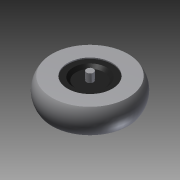
# Autodesk Inventor part: caster wheel
Saved by Autodesk Inventor 2012 (Build 160160000, 160)
## iProperties
Created: 2012-03-07
Part Number: caster wheel
Material: Default
Document SubType Name: Modeling
Designer: esv
Density: 1 g/cm^3
Author: esv
Autodesk Inventor part; units mm, degrees
ref_plane "YZ Plane" through (0, 0, 0) normal (1, 0, 0) x (0, 1, 0)
ref_plane "XZ Plane" through (0, 0, 0) normal (0, 1, 0) x (-1, 0, 0)
ref_plane "XY Plane" through (0, 0, 0) normal (0, 0, 1) x (1, 0, 0)
sketch "Sketch1" plane through (0, 0, 0) normal (0, 0, 1) x (1, 0, 0)
  line L0 (0, 0) -> (0, 0)
  line L1 (95.25, 0) -> (95.25, 7.7978)
  line L2 (86.36, -27.94) -> (50.8, -27.94)
  line L3 (50.8, -27.94) -> (50.8, 27.94)
  line L4 (50.8, 27.94) -> (86.36, 27.94)
  line L5 (86.36, 27.94) -> (86.36, -27.94)
  line L6 (50.8, 25.4) -> (38.1, 25.4)
  line L7 (38.1, 25.4) -> (38.1, -25.4)
  line L8 (38.1, -25.4) -> (50.8, -25.4)
  line L9 (50.8, -25.4) -> (50.8, 25.4)
  line L10 (0, 19.05) -> (31.75, 19.05)
  line L11 (31.75, 19.05) -> (31.75, -19.05)
  line L12 (31.75, -19.05) -> (0, -19.05)
  line L13 (0, -19.05) -> (0, 19.05)
  line L14 (31.75, 19.05) -> (38.1, 25.4)
  line L15 (38.1, -25.4) -> (31.75, -19.05)
  line L16 (0, 7.7978) -> (4.1037, 7.7978)
  line L17 (0, 38.1) -> (7.9375, 38.1)
  line L18 (7.9375, 38.1) -> (7.9375, -38.1)
  line L19 (7.9375, -38.1) -> (0, -38.1)
  line L20 (0, -38.1) -> (0, 38.1)
  arc A0 (86.36, -27.94) -> (86.36, 27.94) centre (46.8993, 0) ccw
  point P0 (50.8, 0)
  point P1 (38.1, 0)
  point P2 (31.75, 0)
  point P3 (50.8, 0)
  dimension "d0" = 95.25
  dimension "d2" = 35.56
  dimension "d3" = 50.8
  dimension "d4" = 50.8
  dimension "d5" = 12.7
  dimension "d6" = 38.1
  dimension "d7" = 6.35
  dimension "d8" = 76.2
  dimension "d9" = 7.9375
  dimension "d10" = 55.88
  constraints: 42 end point, 9 parallel, 7 midpoint, 5 perpendicular, 4 horizontal, 3 horizontal alignment, 2 point on circle, 2 point on line, 1 centre point, 1 collinear, 1 tangent, 1 vertical
  measures "d0" distance between parallel lines of L0 L1
  measures "d2" distance of L3.end L4.end
  measures "d3" distance between parallel lines of L0 L3
  measures "d4" distance between parallel lines of L8 L6
  measures "d5" distance of L6.start L6.end
  measures "d6" distance of L10.end L11.end
  measures "d7" distance between parallel lines of L7 L11
  measures "d8" distance between parallel lines of L19 L17
  measures "d9" distance between parallel lines of L20 L18
  measures "d10" distance between parallel lines of L2 L4
revolve "Revolution1" add sketch "Sketch1" angle 360 about axis through (0, -38.1, 0) along (0, 1, 0)
body "Solid1"
